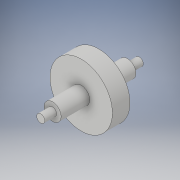
# Autodesk Inventor part: noisemaker
Saved by Autodesk Inventor 2018 (Build 220112000, 112)
## iProperties
Created: 2018-03-09
Part Number: noisemaker
Material: Generic
Document SubType Name: Modeling
Designer: kburke4251
Density: 1 g/cm^3
Appearance: Default
Author: kburke4251
Autodesk Inventor part; units mm, degrees
ref_plane "YZ Plane" through (0, 0, 0) normal (1, 0, 0) x (0, 1, 0)
ref_plane "XZ Plane" through (0, 0, 0) normal (0, 1, 0) x (-1, 0, 0)
ref_plane "XY Plane" through (0, 0, 0) normal (0, 0, 1) x (1, 0, 0)
sketch "Sketch1" plane through (0, 0, 0) normal (0, 0, 1) x (1, 0, 0)
  circle A0 centre (0, 0) radius 0.6731
  dimension "d0" = 1.3462
  constraints: 1 centre point, 1 coincident
  measures "d0" diameter of A0
extrude "Extrusion1" add sketch "Sketch1" against normal blind 1.9812
sketch "Sketch2" plane through (0, 0, -1.9812) normal (0, 0, -1) x (-1, 0, 0)
  circle A0 centre (0, 0) radius 1.4224
  dimension "d3" = 2.8448
  constraints: 1 centre point, 1 coincident
  measures "d3" diameter of A0
extrude "Extrusion2" add sketch "Sketch2" along normal blind 4.8006
sketch "Sketch3" plane through (0, 0, -6.7818) normal (0, 0, -1) x (-1, 0, 0)
  circle A0 centre (0, 0) radius 5.2197
  dimension "d6" = 10.4394
  constraints: 1 centre point, 1 coincident
  measures "d6" diameter of A0
extrude "Extrusion3" add sketch "Sketch3" along normal blind 2.9464
sketch "Sketch4" plane through (0, 0, -9.7282) normal (0, 0, -1) x (-1, 0, 0)
  point P0 (0, 0)
sketch "Sketch5" plane through (0, 0, -9.7282) normal (0, 0, -1) x (-1, 0, 0)
  circle A0 centre (0, 0) radius 1.4224
  dimension "d9" = 2.8448
  constraints: 1 centre point, 1 coincident
  measures "d9" diameter of A0
extrude "Extrusion4" add sketch "Sketch5" along normal blind 4.8006
sketch "Sketch6" plane through (0, 0, -14.5288) normal (0, 0, -1) x (-1, 0, 0)
  circle A0 centre (0, 0) radius 0.6731
  dimension "d12" = 1.3462
  constraints: 1 centre point, 1 coincident
  measures "d12" diameter of A0
extrude "Extrusion5" add sketch "Sketch6" along normal blind 1.9812
body "Solid1"
